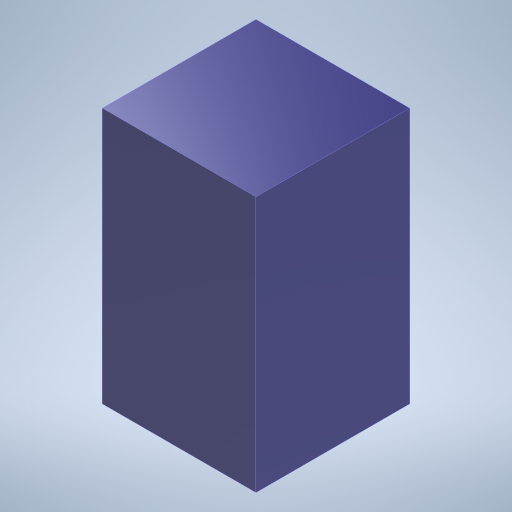
# Autodesk Inventor part: DISTANCE_BRICK_SIDE
Saved by Autodesk Inventor 2023 (Build 270158000, 158)
## iProperties
Created: 2024-02-22
Part Number: DISTANCE_BRICK_SIDE
Material: Wood (Birch)
Document SubType Name: Modeling
Designer: vraco
Density: 0.55 g/cm^3
Appearance: Flaked Satin - Dark Blue
Author: vraco
Autodesk Inventor part; units mm, degrees
ref_plane "YZ Plane" through (0, 0, 0) normal (1, 0, 0) x (0, 1, 0)
ref_plane "XZ Plane" through (0, 0, 0) normal (0, 1, 0) x (-1, 0, 0)
ref_plane "XY Plane" through (0, 0, 0) normal (0, 0, 1) x (1, 0, 0)
sketch "Sketch1" plane through (0, 0, 0) normal (0, 1, 0) x (-1, 0, 0)
  line L0 (0, -21) -> (0, 21) projected
  line L1 (-21, 0) -> (21, 0) projected
  line L2 (15, 15) -> (-15, 15)
  line L3 (-15, 15) -> (-15, -15)
  line L4 (-15, -15) -> (15, -15)
  line L5 (15, -15) -> (15, 15)
  point P0 (0, 0)
  dimension "d0" = 30
  dimension "d1" = 30
  constraints: 8 end point, 2 parallel, 1 horizontal, 1 perpendicular, 2 other
  measures "d0" distance of L4.end L2.start
  measures "d1" distance of L3.end L4.end
extrude "Extrusion1" add sketch "Sketch1" along normal blind 50
equation "\"d1\" = d0"
body "Solid1"
